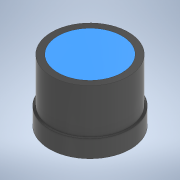
# Autodesk Inventor part: NikkonTubelens
Saved by Autodesk Inventor 2020 (Build 240168000, 168)
## iProperties
Created: 2019-08-07
Part Number: NikkonTubelens
Material: Generic
Document SubType Name: Modeling
Designer: Julian
Density: 1 g/cm^3
Appearance: Default
Author: Julian
Autodesk Inventor part; units mm, degrees
ref_plane "YZ Plane" through (0, 0, 0) normal (1, 0, 0) x (0, 1, 0)
ref_plane "XZ Plane" through (0, 0, 0) normal (0, 1, 0) x (-1, 0, 0)
ref_plane "XY Plane" through (0, 0, 0) normal (0, 0, 1) x (1, 0, 0)
sketch "Sketch1" plane through (0, 0, 0) normal (0, 1, 0) x (-1, 0, 0)
  circle A0 centre (0, 0) radius 19
  circle A1 centre (0, 0) radius 18
  circle A2 centre (0, 0) radius 15
  dimension "d0" = 38
  dimension "d1" = 36
  dimension "d2" = 30
  constraints: 3 centre point, 3 coincident
  measures "d0" diameter of A0
  measures "d1" diameter of A1
  measures "d2" diameter of A2
extrude "Extrusion1" add sketch "Sketch1" along normal blind 29 contours A1
extrude "Extrusion2" add sketch "Sketch1" along normal blind 8.15 contours A0
extrude "Extrusion3" add sketch "Sketch1" along normal blind 29.001 contours A2
extrude "Extrusion4" add sketch "Sketch1" against normal blind 0.001 contours A2
body "Solid1"
